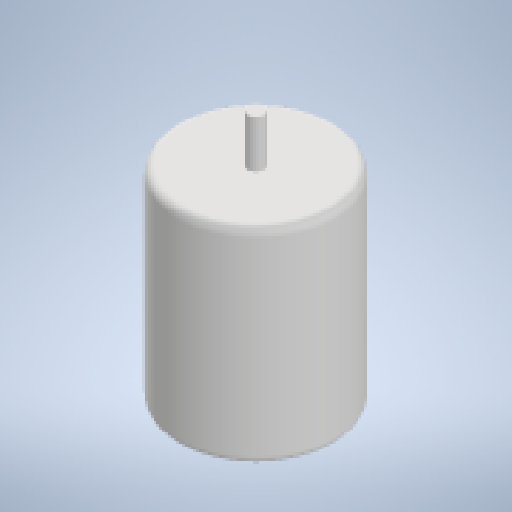
# Autodesk Inventor part: МоторКолес
Saved by Autodesk Inventor 2024.2 (Build 282272000, 272)
## iProperties
Created: 2025-03-04
Part Number: МоторКолес
Material: Типовые
Document SubType Name: Modeling
Designer: Timofey
Density: 1 g/cm^3
Appearance: По умолчанию
Mass: 1020.08 g
Surface Area: 561.205 cm^2
Volume: 1020.08 cm^3
Author: Timofey
Autodesk Inventor part; units mm, degrees
ref_plane "YZ Plane" through (0, 0, 0) normal (1, 0, 0) x (0, 1, 0)
ref_plane "XZ Plane" through (0, 0, 0) normal (0, 1, 0) x (-1, 0, 0)
ref_plane "XY Plane" through (0, 0, 0) normal (0, 0, 1) x (1, 0, 0)
sketch "Эскиз1" plane through (0, 0, 0) normal (0, 1, 0) x (-1, 0, 0)
  circle A0 centre (0, 0) radius 50
  dimension "d0" = 100
  constraints: 1 centre point, 1 coincident
  measures "d0" diameter of A0
extrude "Выдавливание1" add sketch "Эскиз1" along normal blind 130
sketch "Эскиз2" plane through (0, 130, 0) normal (0, 1, 0) x (1, 0, 0)
  circle A0 centre (0, 0) radius 5
  dimension "d3" = 10
  constraints: 1 centre point, 1 coincident
  measures "d3" diameter of A0
extrude "Выдавливание2" add sketch "Эскиз2" along normal blind 30
fillet "Сопряжение1" radius 5 2 edges at (50, 130, 0) (50, 0, 0)
